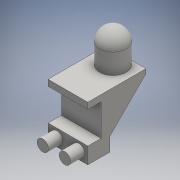
# Autodesk Inventor part: SLP3
Saved by Autodesk Inventor 2016 (Build 200138000, 138)
## iProperties
Created: 2018-03-26
Part Number: SLP3
Material: Generic
Document SubType Name: Modeling
Designer: Tyler
Density: 1 g/cm^3
Appearance: Default
Author: Tyler
Autodesk Inventor part; units mm, degrees
ref_plane "YZ Plane" through (0, 0, 0) normal (1, 0, 0) x (0, 1, 0)
ref_plane "XZ Plane" through (0, 0, 0) normal (0, 1, 0) x (-1, 0, 0)
ref_plane "XY Plane" through (0, 0, 0) normal (0, 0, 1) x (1, 0, 0)
sketch "Sketch1" plane through (0, 0, 0) normal (1, 0, 0) x (0, 1, 0)
  line L0 (0, 5.2) -> (6.6, 5.2)
  line L1 (6.6, 5.2) -> (6.6, 4.7)
  line L2 (2.5, 0.6) -> (2.5, -0.9618)
  line L3 (2.5, -0.9618) -> (0, -0.9618)
  line L4 (0, -0.9618) -> (0, 0.9)
  line L5 (0, 0.9) -> (1.5, 0.9)
  line L6 (1.5, 0.9) -> (1.5, 4.5)
  line L7 (1.5, 4.5) -> (0, 4.5)
  line L8 (0, 4.5) -> (0, 5.2)
  line L9 (6.6, 4.7) -> (2.5, 0.6)
  point P0 (0, 0)
  point P1 (1.5, 2.7)
  point P2 (0, 0)
  dimension "d0" = 3.6
  dimension "d1" = 1.5
  dimension "d2" = 6.6
  dimension "d3" = 45
  dimension "d4" = 5.2
  dimension "d6" = 2.7
  dimension "d7" = 0
  dimension "d8" = 1
  dimension "d9" = 0.5
  constraints: 20 end point, 7 perpendicular, 2 point on line, 1 horizontal, 1 midpoint, 1 parallel
  measures "d0" distance between parallel lines of L5 L7
  measures "d1" distance between parallel lines of L4 L6
  measures "d2" distance between parallel lines of L8 L1
  measures "d3" angle of L9 L1
  measures "d4" distance from line of point (0, 0) L0
  measures "d6" vertical distance of point (0, 0) point (1.5, 2.7)
  measures "d7" distance of point (0, 0) point (0, 0)
  measures "d8" distance between parallel lines of L6 L2
  measures "d9" distance of L0.end L1.end
extrude "Extrusion1" add sketch "Sketch1" along normal mid plane 4.5
sketch "Sketch2" plane through (-2.25, 0, 5.2) normal (0, 0, 1) x (1, 0, 0)
  line L0 (2.25, 0) -> (2.25, 10.2) construction
  circle A0 centre (2.25, 5.1) radius 1.5
  line L1 (4.5, 6.6) -> (0, 6.6) projected
  dimension "d12" = 3
  constraints: 2 end point, 1 centre point, 1 midpoint, 1 tangent, 1 vertical
  measures "d12" diameter of A0
extrude "Extrusion2" add sketch "Sketch2" along normal blind 3.8
fillet "Fillet1" radius 1.5 1 edges at (-1.5, 5.1, 9)
sketch "Sketch3" plane through (-2.25, 0, -0.9618) normal (0, -1, 0) x (1, 0, 0)
  circle A0 centre (1, 0.9618) radius 0.65
  circle A1 centre (3.5, 0.9618) radius 0.65
  line L0 (0, 6.1618) -> (4.5, 6.1618) projected
  point P0 (2.25, 0.9618)
  dimension "d16" = 1.3
  dimension "d17" = 1.3
  dimension "d18" = 5.2
  dimension "d19" = 1.25
  dimension "d20" = 1.25
  dimension "d21" = 5.2
  constraints: 2 centre point
  measures "d16" diameter of A0
  measures "d17" diameter of A1
  measures "d18" distance from line of A0.centre L0
  measures "d19" distance of A0.centre point (2.25, 0.962)
  measures "d20" distance of point (2.25, 0.962) A1.centre
  measures "d21" distance from line of L0 A1.centre
extrude "Extrusion3" add sketch "Sketch3" along normal blind 1.6
body "Solid1"
